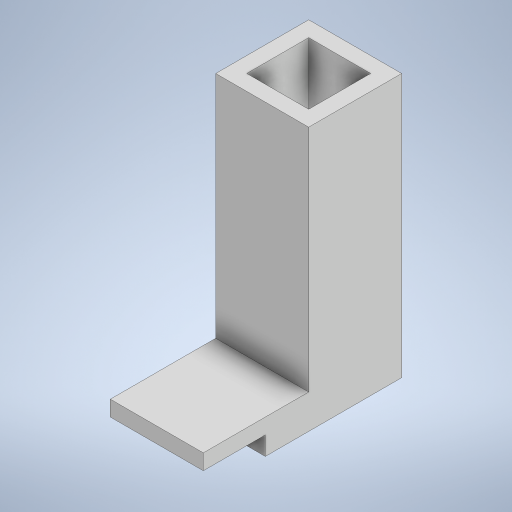
# Autodesk Inventor part: flexibler_standfuß_v0.5
Saved by Autodesk Inventor 2024 (Build 280153000, 153)
## iProperties
Created: 2023-12-27
Part Number: flexibler_standfuß_v0.5
Material: Generic
Document SubType Name: Modeling
Designer: Julian
Density: 1 g/cm^3
Appearance: Default
Author: Julian
Autodesk Inventor part; units mm, degrees
ref_plane "YZ Plane" through (0, 0, 0) normal (1, 0, 0) x (0, 1, 0)
ref_plane "XZ Plane" through (0, 0, 0) normal (0, 1, 0) x (-1, 0, 0)
ref_plane "XY Plane" through (0, 0, 0) normal (0, 0, 1) x (1, 0, 0)
sketch "Sketch1" plane through (0, 0, 0) normal (1, 0, 0) x (0, 1, 0)
  line L0 (0, 0) -> (0, -30)
  line L1 (11, 0) -> (30, 0) construction
  line L2 (0, -30) -> (85, -30)
  line L3 (11, 0) -> (85, 0)
  line L4 (85, 0) -> (85, -30)
  line L5 (0, 0) -> (0, 14)
  line L6 (11, 0) -> (14, 0) construction
  line L7 (0, 14) -> (6, 14)
  line L8 (6, 14) -> (6, 34)
  line L9 (6, 34) -> (11, 34)
  line L10 (11, 34) -> (11, 0)
  dimension "d0" = 30
  dimension "d2" = 85
  dimension "d4" = 14
  dimension "d6" = 6
  dimension "d7" = 20
  dimension "d8" = 5
  dimension "d9" = 34
  constraints: 22 end point, 4 horizontal, 4 vertical, 1 perpendicular, 1 point on line
  measures "d0" distance of L0.start L0.end
  measures "d2" distance of L0.end L2.end
  measures "d4" distance of L0.start L5.end
  measures "d6" distance of L5.end L7.end
  measures "d7" distance of L7.end L8.end
  measures "d8" distance of L8.end L9.end
  measures "d9" distance of L1.start L9.end
extrude "Extrusion1" add sketch "Sketch1" along normal blind 30
sketch "Sketch2" plane through (0, 85, 0) normal (0, 1, 0) x (1, 0, 0)
  line L0 (5, 5) -> (5, 25)
  line L1 (5, 5) -> (25, 5) construction
  line L2 (5, 25) -> (25, 25)
  line L3 (25, 25) -> (25, 5)
  line L4 (25, 5) -> (5, 5)
  point P0 (0, 0)
  dimension "d13" = 20
  dimension "d14" = 90
  dimension "d15" = 20
  dimension "d16" = 90
  dimension "d17" = 20
  dimension "d18" = 90
  dimension "d19" = 20
  dimension "d20" = 90
  constraints: 10 end point, 3 perpendicular, 1 horizontal, 1 vertical
  measures "d13" distance of L0.start L0.end
  measures "d14" angle of L1 L0
  measures "d15" distance of L0.end L2.end
  measures "d16" angle of L0 L2
  measures "d17" distance of L2.end L3.end
  measures "d18" angle of L2 L3
  measures "d19" distance of L3.end L0.start
  measures "d20" angle of L3 L4
extrude "Extrusion2" cut sketch "Sketch2" against normal blind 80
sketch "Sketch3" plane through (0, 0, 0) normal (-1, 0, 0) x (0, 0, 1)
  point P0 (0, 0)
body "Solid1"
